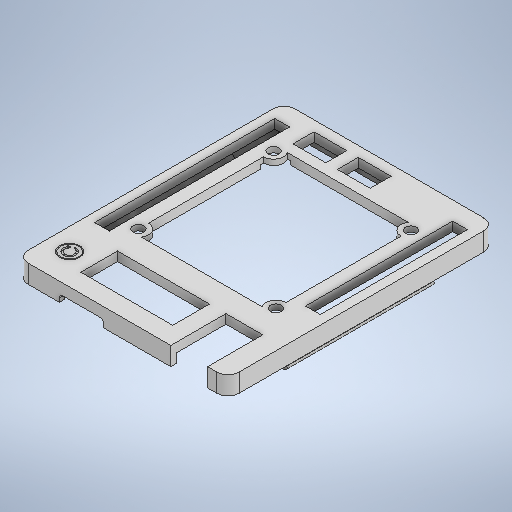
# Autodesk Inventor part: uno_r4_lid
Saved by Autodesk Inventor 2025.2 (Build 292293000, 293)
## iProperties
Created: 2025-03-24
Part Number: uno_r4_lid
Material: Generic
Document SubType Name: Modeling
Designer: caomi
Density: 1 g/cm^3
Appearance: Default
Author: caomi
Autodesk Inventor part; units mm, degrees
sketch "Sketch1" plane through (0, 0, 0) normal (0, 1, 0) x (-1, 0, 0)
  line L0 (0, 0) -> (53.34, 0) construction
  line L1 (53.34, 0) -> (53.34, -68.58) construction
  line L2 (53.34, -68.58) -> (0, -68.58) construction
  line L3 (0, -68.58) -> (0, 0) construction
  line L4 (55.34, -70.58) -> (55.34, 2)
  line L5 (55.34, 2) -> (-2, 2)
  line L6 (-2, 2) -> (-2, -70.58)
  line L7 (-2, -70.58) -> (55.34, -70.58)
  dimension "d0" = 53.34
  dimension "d1" = 68.58
  dimension "d2" = 2
  constraints: 16 end point, 4 parallel, 2 perpendicular, 1 horizontal, 3 other
  measures "d0" distance of L0.start L0.end
  measures "d1" distance of L2.end L0.start
  measures "d2" distance between parallel lines of L1 L4
extrude "Body" add sketch "Sketch1" against normal blind 5
fillet "Fillet1" radius 3 4 edges at (-55.34, -2.5, 2) (-55.34, -2.5, -70.58) (2, -2.5, -70.58) (2, -2.5, 2)
shell "Shell1" thickness 1.5 removed faces 1 at (-17.1133, -5, -45.3867)
sketch "Sketch2" plane through (0, -5, 0) normal (0, -1, 0) x (1, 0, 0)
  line L0 (-53.34, 0) -> (-53.34, -68.58) construction
  line L1 (-52.34, 0.5) -> (-1, 0.5) projected
  line L2 (-1, 2) -> (-52.34, 2) projected
  line L3 (-43.84, 0.5) -> (-31.84, 0.5)
  line L4 (-31.84, 0.5) -> (-31.84, 2)
  line L5 (-31.84, 2) -> (-43.84, 2)
  line L6 (-43.84, 2) -> (-43.84, 0.5)
  line L7 (-13.54, 2) -> (-3.54, 2)
  line L8 (-3.54, 2) -> (-3.54, -13)
  line L9 (-3.54, -13) -> (-13.54, -13)
  line L10 (-13.54, -13) -> (-13.54, 2)
  dimension "d8" = 12
  dimension "d15" = 9.5
  dimension "d16" = 39.8
  dimension "d17" = 10
  dimension "d18" = 15
  constraints: 16 end point, 4 parallel, 3 point on line, 2 horizontal, 2 perpendicular
  measures "d8" distance between parallel lines of L4 L6
  measures "d15" distance from line of L0 L5.end
  measures "d16" distance between parallel lines of L0 L10
  measures "d17" distance between parallel lines of L8 L10
  measures "d18" distance of L9.end L7.start
extrude "USB-C port" cut sketch "Sketch2" against normal blind 2 contours L6 L2 L4 L1
fillet "Fillet2" radius 1 2 edges at (-43.84, -3, 1.25) (-31.84, -3, 1.25)
extrude "DC jack port" cut sketch "Sketch2" against normal through all contours L10 L2 L8 L1 | L1 L8 L9 L10
sketch "Sketch3" plane through (0, 0, 0) normal (0, 1, 0) x (1, 0, 0)
  line L0 (-53.34, 0) -> (-53.34, 68.58) construction
  line L1 (-52.84, 65.58) -> (-48.84, 65.58)
  line L2 (-48.84, 65.58) -> (-48.84, 16.58)
  line L3 (-48.84, 16.58) -> (-52.84, 16.58)
  line L4 (-52.84, 16.58) -> (-52.84, 65.58)
  line L5 (-53.34, 68.58) -> (0, 68.58) construction
  line L6 (-0.5, 65.58) -> (-4.5, 65.58)
  line L7 (-4.5, 65.58) -> (-4.5, 25.58)
  line L8 (-4.5, 25.58) -> (-0.5, 25.58)
  line L9 (-0.5, 25.58) -> (-0.5, 65.58)
  line L10 (0, 68.58) -> (0, 0) construction
  line L11 (-32.34, 67.78) -> (-23.44, 67.78)
  line L12 (-23.44, 67.78) -> (-23.44, 62.08)
  line L13 (-23.44, 62.08) -> (-32.34, 62.08)
  line L14 (-32.34, 62.08) -> (-32.34, 67.78)
  dimension "d19" = 0.5
  dimension "d20" = 4
  dimension "d23" = 3
  dimension "d24" = 52
  dimension "d25" = 0.5
  dimension "d26" = 3
  dimension "d27" = 40
  dimension "d28" = 21
  dimension "d29" = 8.9
  dimension "d30" = 5.7
  dimension "d31" = 0.8
  constraints: 24 end point, 6 parallel, 3 horizontal, 3 perpendicular, 1 collinear
  measures "d19" distance between parallel lines of L0 L4
  measures "d20" distance of L2.end L3.end
  measures "d23" distance between parallel lines of L5 L1
  measures "d24" distance between parallel lines of L3 L5
  measures "d25" distance between parallel lines of L10 L9
  measures "d26" distance from line of L5 L6.start
  measures "d27" distance of L8.end L6.start
  measures "d28" distance from line of L0 L11.start
  measures "d29" distance of L11.start L11.end
  measures "d30" distance of L13.end L11.start
  measures "d31" vertical distance of L0.end L11.start
extrude "GPIO cutouts" cut sketch "Sketch3" against normal blind 5
sketch "Sketch4" plane through (0, 0, 0) normal (0, 1, 0) x (1, 0, 0)
  line L0 (-48.17, 60.8905) -> (-5.17, 60.8905) construction
  line L1 (-5.17, 60.8905) -> (-5.17, 17.8905) construction
  line L2 (-5.17, 17.8905) -> (-48.17, 17.8905) construction
  line L3 (-48.17, 17.8905) -> (-48.17, 60.8905) construction
  line L4 (-48.17, 60.8905) -> (-5.17, 17.8905) construction
  line L5 (-5.17, 60.8905) -> (-48.17, 17.8905) construction
  line L6 (-45.36, 57.7615) -> (-7.98, 57.7615) construction
  line L7 (-7.98, 57.7615) -> (-7.98, 21.0195) construction
  line L8 (-7.98, 21.0195) -> (-45.36, 21.0195) construction
  line L9 (-45.36, 21.0195) -> (-45.36, 57.7615) construction
  line L10 (-45.36, 57.7615) -> (-7.98, 21.0195) construction
  line L11 (-7.98, 57.7615) -> (-45.36, 21.0195) construction
  circle A0 centre (-7.98, 21.0195) radius 1.5
  circle A1 centre (-45.36, 21.0195) radius 1.5
  circle A2 centre (-45.36, 57.7615) radius 1.5
  circle A3 centre (-7.98, 57.7615) radius 1.5
  circle A4 centre (-7.98, 21.0195) radius 2.75
  circle A5 centre (-45.36, 21.0195) radius 2.75
  circle A6 centre (-7.98, 57.7615) radius 2.75
  circle A7 centre (-45.36, 57.7615) radius 2.75
  line L12 (-10.73, 21.0195) -> (-42.61, 21.0195)
  line L13 (-45.36, 23.7695) -> (-45.36, 55.0115)
  line L14 (-42.61, 57.7615) -> (-10.73, 57.7615)
  line L15 (-7.98, 23.7695) -> (-7.98, 55.0115)
  line L16 (-4.5, 65.58) -> (-0.5, 65.58) projected
  line L17 (-48.84, 65.58) -> (-4.5, 65.58) construction
  line L18 (-43.0551, 59.2615) -> (-10.2849, 59.2615)
  line L19 (-43.0551, 19.5195) -> (-10.2849, 19.5195)
  point P0 (-26.67, 39.3905)
  point P1 (-26.67, 65.58)
  dimension "d34" = 43
  dimension "d35" = 37.38
  dimension "d36" = 36.742
  dimension "d37" = 3
  dimension "d43" = 5.5
  dimension "d101" = 1.5
  dimension "d102" = 1.5
  constraints: 38 end point, 12 point on circle, 8 centre point, 8 coincident, 7 point on line, 6 equal radius, 6 parallel, 5 midpoint, 3 collinear, 3 perpendicular, 2 horizontal, 1 vertical alignment
  measures "d34" distance of L1.end L2.end
  measures "d35" distance of L7.end L8.end
  measures "d36" distance of L8.end L6.start
  measures "d37" diameter of A0
  measures "d43" diameter of A4
  measures "d101" distance between parallel lines of L14 L18
  measures "d102" distance between parallel lines of L12 L19
sketch "Sketch7" plane through (-52.34, -1.5, -69.08) normal (0, -1, 0) x (1, 0, 0)
  line L0 (3.5, 52.5) -> (3.5, 3.5) projected
  line L1 (3.5, 3.5) -> (-0.5, 3.5) projected
  line L2 (-0.5, 3.5) -> (-0.5, 52.5) projected
  line L3 (-0.5, 52.5) -> (3.5, 52.5) projected
  line L4 (47.84, 43.5) -> (51.84, 43.5) projected
  line L5 (51.84, 43.5) -> (51.84, 3.5) projected
  line L6 (51.84, 3.5) -> (47.84, 3.5) projected
  line L7 (47.84, 3.5) -> (47.84, 43.5) projected
  line L8 (28.9, 7) -> (28.9, 1.3) projected
  line L9 (28.9, 1.3) -> (20, 1.3) projected
  line L10 (20, 1.3) -> (20, 7) projected
  line L11 (20, 7) -> (28.9, 7) projected
  line L12 (48.8, 69.58) -> (48.8, 56.08) projected
  line L13 (48.8, 56.08) -> (38.8, 56.08) projected
  line L14 (38.8, 56.08) -> (38.8, 69.58) projected
  line L15 (0, 69.58) -> (38.8, 69.58) projected
  arc A0 (0, 69.58) -> (-1.5, 68.08) centre (0, 68.08) ccw projected
  line L16 (-1.5, 1.5) -> (-1.5, 68.08) projected
  arc A1 (-1.5, 1.5) -> (0, 0) centre (0, 1.5) ccw projected
  line L17 (51.34, 0) -> (0, 0) projected
  arc A2 (51.34, 0) -> (52.84, 1.5) centre (51.34, 1.5) ccw projected
  line L18 (52.84, 68.08) -> (52.84, 1.5) projected
  arc A3 (52.84, 68.08) -> (51.34, 69.58) centre (51.34, 68.08) ccw projected
  line L19 (48.8, 69.58) -> (51.34, 69.58) projected
  point P0 (52.34, 69.08)
extrude "Thicken the top" add sketch "Sketch7" along normal blind 1
extrude "Screw hole motor driver" cut sketch "Sketch4" against normal through all contours A0 | A1 | A2 | A3
sketch "Sketch5" plane through (-52.34, -2.5, -69.08) normal (0, -1, 0) x (1, 0, 0)
  line L0 (47.51, 46.2419) -> (44.36, 44.4232)
  line L1 (44.36, 44.4232) -> (41.21, 46.2419)
  line L2 (41.21, 46.2419) -> (41.21, 49.8792)
  line L3 (41.21, 49.8792) -> (44.36, 51.6978)
  line L4 (44.36, 51.6978) -> (47.51, 49.8792)
  line L5 (47.51, 49.8792) -> (47.51, 46.2419)
  line L6 (47.51, 13.1372) -> (47.51, 9.4999)
  line L7 (47.51, 9.4999) -> (44.36, 7.6812)
  line L8 (44.36, 7.6812) -> (41.21, 9.4999)
  line L9 (41.21, 9.4999) -> (41.21, 13.1372)
  line L10 (41.21, 13.1372) -> (44.36, 14.9558)
  line L11 (44.36, 14.9558) -> (47.51, 13.1372)
  circle A0 centre (6.98, 48.0605) radius 1.5 projected
  line L12 (10.13, 49.8792) -> (10.13, 46.2419)
  line L13 (10.13, 46.2419) -> (6.98, 44.4232)
  line L14 (6.98, 44.4232) -> (3.83, 46.2419)
  line L15 (3.83, 46.2419) -> (3.83, 49.8792)
  line L16 (3.83, 49.8792) -> (6.98, 51.6978)
  line L17 (6.98, 51.6978) -> (10.13, 49.8792)
  line L18 (10.13, 13.1372) -> (10.13, 9.4999)
  line L19 (10.13, 9.4999) -> (6.98, 7.6812)
  line L20 (6.98, 7.6812) -> (3.83, 9.4999)
  line L21 (3.83, 9.4999) -> (3.83, 13.1372)
  line L22 (3.83, 13.1372) -> (6.98, 14.9558)
  line L23 (6.98, 14.9558) -> (10.13, 13.1372)
  circle A1 centre (6.98, 11.3185) radius 1.5 projected
  circle A2 centre (44.36, 11.3185) radius 1.5 projected
  circle A3 centre (44.36, 48.0605) radius 1.5 projected
  circle A4 centre (6.98, 48.0605) radius 1.5 projected
  dimension "d40" = 6.3
  constraints: 48 end point, 5 coincident, 4 vertical, 3 equal length, 52 other
  measures "d40" distance between parallel lines of L2 L5
extrude "M3 nut slot" cut sketch "Sketch5" against normal blind 1 contours L0 L1 L2 L3 L4 L5 | L6 L7 L8 L9 L10 L11 | L12 L13 L14 L15 L16 L17 | L18 L19 L20 L21 L22 L23 | A1 | A2 | A3
extrude "Recess face motor driver" cut sketch "Sketch4" against normal blind 3 contours A4 L12 A5 L13 A7 L14 A6 L15 | L19 A5 L12 A4 | L14 A7 L18 A6
ref_plane "Work Plane1" through (0, 0, -15) normal (0, 0, 1) x (1, 0, 0)
ref_plane "Work Plane2" through (0, 0, -55) normal (0, 0, 1) x (1, 0, 0)
sketch "Sketch8" plane through (0, 0, -15) normal (0, 0, 1) x (1, 0, 0)
  line L0 (-53.84, -3.5) -> (-52.64, -4.7)
  line L1 (-52.64, -4.7) -> (-52.64, -7.3)
  line L2 (-52.64, -7.3) -> (-53.84, -7.3)
  line L3 (-53.84, -7.3) -> (-53.84, -3.5)
  line L4 (-53.84, -2.5) -> (-53.84, -5) projected
  line L5 (-53.84, -5.7) -> (-54.64, -6.5)
  line L6 (-54.64, -6.5) -> (-53.84, -7.3)
  line L7 (-54.64, -6.5) -> (-53.84, -6.5) construction
  point P0 (0, 0)
  point P1 (-53.84, -7.5)
  dimension "d53" = 1.5
  dimension "d54" = 45
  dimension "d56" = 1.2
  dimension "d57" = 45
  dimension "d58" = 0.8
  dimension "d62" = 1.5
  constraints: 15 end point, 2 perpendicular, 2 point on line, 2 vertical, 1 collinear, 1 other
  measures "d53" distance of L4.end L0.start
  measures "d54" angle of L0 L4
  measures "d56" distance of L2.end L1.end
  measures "d57" angle of L3 L6
  measures "d58" distance of L5.end L7.end
  measures "d62" distance from line of L4.end L7
extrude "Snap tab 1" add sketch "Sketch8" against normal up to surface (40 mm away)
fillet "Fillet3" radius 0.5 1 edges at (-54.64, -6.5, -35)
ref_plane "Work Plane3" through (-26.67, 0, -67.58) normal (-1, 0, 0) x (0, 0, 1)
mirror "Snap tab right side" about plane through (-26.67, 0, -67.58) normal (-1, 0, 0) of "Snap tab 1", "Fillet3"
sketch "Sketch9" plane through (-52.34, -2.5, -69.08) normal (0, -1, 0) x (1, 0, 0)
  line L0 (52.34, 69.08) -> (-1, 69.08) construction
  line L1 (-1, 69.08) -> (-1, 0.5) construction
  circle A0 centre (2.937, 62.73) radius 2.5
  circle A1 centre (2.937, 62.73) radius 2.75
  dimension "d66" = 6.35
  dimension "d67" = 3.937
  dimension "d71" = 5
  dimension "d73" = 5.5
  constraints: 2 centre point, 2 coincident
  measures "d66" distance from line of L0 point (2.937, 62.73)
  measures "d67" distance from line of L1 point (2.937, 62.73)
  measures "d71" diameter of A0
  measures "d73" diameter of A1
extrude "Extrusion12" cut sketch "Sketch9" against normal through all contours A0 | A1
extrude "Reset button" add sketch "Sketch9" along normal blind 3 and the other way blind 2.5 separate body contours A0
ref_plane "Work Plane5" through (-49.403, -2.5, -6.35) normal (0, 0, 1) x (1, 0, 0)
ref_plane "Work Plane4" through (-49.403, -2.5, -8.85) normal (0, 0, 1) x (1, 0, 0)
sketch "Sketch10" plane through (-49.403, -2.5, -6.35) normal (0, 0, 1) x (1, 0, 0)
  line L0 (-2.5, 2.5) -> (-2.5, -3) projected
  line L1 (-2.5, -2.1) -> (-3.3, -1.3)
  line L2 (-3.3, -1.3) -> (-2.5, -0.5)
  line L3 (-3.3, -1.3) -> (-2.5, -1.3) construction
  line L4 (2.75, 0) -> (-2.75, 0) projected
  line L5 (-2.75, 0) -> (-2.75, 0.65)
  line L6 (-2.75, 0.65) -> (-3.7, -0.3)
  line L7 (-2.75, -2.25) -> (-2.75, -3.25)
  line L8 (-4.25, -3.25) -> (-4.25, 0)
  line L9 (-3.7, -0.3) -> (-3.7, -1.3)
  line L10 (-3.7, -1.3) -> (-2.75, -2.25)
  line L11 (-2.75, 0) -> (-4.25, 0)
  line L12 (-2.5, -2.1) -> (-2.5, -0.5)
  line L13 (-2.5, -3) -> (2.5, -3) projected
  line L14 (0, -4.6511) -> (0, -1.8) construction
  line L15 (-4.25, -3.25) -> (-2.75, -3.25)
  point P0 (49.403, 2.5)
  point P1 (0, -3)
  point P2 (-3.4, 0)
  dimension "d79" = 45
  dimension "d80" = 0.8
  dimension "d81" = 0.5
  dimension "d82" = 135
  dimension "d83" = 1
  dimension "d85" = 1.5
  dimension "d90" = 1
  dimension "d98" = 0.4
  constraints: 26 end point, 5 point on line, 5 vertical, 2 collinear, 2 horizontal, 1 midpoint, 1 parallel, 1 perpendicular, 1 other
  measures "d79" angle of L0 L2
  measures "d80" distance of L1.end L3.end
  measures "d81" vertical distance of L2.end L4.end
  measures "d82" angle of L5 L6
  measures "d83" distance of L6.end L9.end
  measures "d85" distance from line of L4.end L8
  measures "d90" distance of L7.start L7.end
  measures "d98" distance from line of L1.end L9
revolve "Revolution1" add sketch "Sketch10" angle 360 about axis through (-49.403, -7.1511, -6.35) along (0, 1, 0) bodies 2 contours L0 L1 L2
revolve "Revolution3" cut sketch "Sketch10" angle 360 about axis through (-49.403, -7.1511, -6.35) along (0, 1, 0) bodies 1 contours L11 L6 L5
revolve "Revolution2" add sketch "Sketch10" angle 360 about axis through (-49.403, -7.1511, -6.35) along (0, 1, 0) bodies 1 contours L6 L9 L10 L7 L15 L8 L11
fillet "Fillet5" radius 1 1 edges at (-45.153, -5.75, -6.35)
ref_plane "Work Plane6" through (-49.403, 0.5, -6.35) normal (0, 1, 0) x (1, 0, 0)
sketch "Sketch11" plane through (-49.403, 0, -6.35) normal (0, 1, 0) x (1, 0, 0)
  arc A0 (-1.0607, 1.0607) -> (0, 1.5) centre (0, 0) ccw construction
  arc A1 (-1.2021, 1.2021) -> (0, 1.7) centre (0, 0) ccw
  arc A2 (-0.9192, 0.9192) -> (0, 1.3) centre (0, 0) ccw
  arc A3 (-0.9192, 0.9192) -> (-1.2021, 1.2021) centre (-1.0607, 1.0607) ccw
  arc A4 (0, 1.7) -> (0, 1.3) centre (0, 1.5) ccw
  line L0 (0, 0) -> (-1.0607, 1.0607) construction
  line L1 (0, 0) -> (0, 1.5) construction
  line L2 (-1.0607, 1.0607) -> (-1.5607, 1.0607) construction
  line L3 (-1.0607, 1.2607) -> (-1.5607, 1.2607)
  line L4 (-1.5607, 0.8607) -> (-1.0607, 0.8607)
  arc A5 (-1.0607, 0.8607) -> (-1.0607, 1.2607) centre (-1.0607, 1.0607) ccw
  arc A6 (-1.5607, 1.2607) -> (-1.5607, 0.8607) centre (-1.5607, 1.0607) ccw
  line L5 (-1.0607, 1.0607) -> (-1.0607, 0.5607) construction
  line L6 (-1.2607, 1.0607) -> (-1.2607, 0.5607)
  line L7 (-0.8607, 0.5607) -> (-0.8607, 1.0607)
  arc A7 (-0.8607, 1.0607) -> (-1.2607, 1.0607) centre (-1.0607, 1.0607) ccw
  arc A8 (-1.2607, 0.5607) -> (-0.8607, 0.5607) centre (-1.0607, 0.5607) ccw
  circle A9 centre (0, 0) radius 2.5 projected
  point P0 (49.403, -6.35)
  point P1 (-1.3107, 1.0607)
  point P2 (-1.0607, 0.8107)
  point P3 (-1.466, 0.8607)
  point P4 (-1.2223, 0.4428)
  point P5 (-0.8607, 1.0607)
  point P6 (-1.0607, 1.2607)
  dimension "d91" = 1.5
  dimension "d92" = 45
  dimension "d93" = 0.4
  dimension "d94" = 0.5
  dimension "d95" = 0.5
  constraints: 20 end point, 19 point on circle, 12 tangent, 9 centre point, 2 concentric, 2 midpoint, 2 parallel, 1 coincident, 1 horizontal, 1 perpendicular, 1 vertical
  measures "d91" radius of A0
  measures "d92" angle of L1 L0
  measures "d93" diameter of A3
  measures "d94" distance of L0.end L2.end
  measures "d95" distance of L0.end L5.end
extrude "Extrusion14" cut sketch "Sketch11" against normal blind 0.5 contours A7 L6 L4 A1 | A1 L4 A6 L3 A3 | A3 A5 L4 L6 A7 | L4 L6 A8 A2 A4 A1 | L4 A5 A2 A8 L6 | L7 A8 A2 A3 bodies 2
fillet "Fillet6" radius 0.5 1 edges at (-46.103, -3.8, -6.35)
sketch "Sketch12" plane through (0, 0, 0) normal (0, 1, 0) x (1, 0, 0)
  line L0 (-43.0261, 13) -> (-18.0261, 13)
  line L1 (-18.0261, 13) -> (-18.0261, 3)
  line L2 (-18.0261, 3) -> (-43.0261, 3)
  line L3 (-43.0261, 3) -> (-43.0261, 13)
  line L4 (-13.54, 13) -> (-3.54, 13) projected
  line L5 (-35.4833, 62.08) -> (-44.3833, 62.08)
  line L6 (-44.3833, 62.08) -> (-44.3833, 67.78)
  line L7 (-44.3833, 67.78) -> (-35.4833, 67.78)
  line L8 (-35.4833, 67.78) -> (-35.4833, 62.08)
  line L9 (-23.44, 62.08) -> (-32.34, 62.08) projected
  line L10 (-32.34, 67.78) -> (-23.44, 67.78) projected
  point P0 (0, 0)
  dimension "d105" = 10
  dimension "d106" = 25
  constraints: 16 end point, 4 collinear, 4 parallel, 2 horizontal, 2 perpendicular
  measures "d105" distance of L2.end L0.start
  measures "d106" distance of L1.end L2.end
extrude "Extrusion15" cut sketch "Sketch12" against normal blind 3 bodies 1
equation "\"d2\" = base_wall + tolerance_general"
equation "\"d6\" = base_wall"
equation "\"uno_width\" = 53.34"
equation "\"uno_length\" = 68.58"
equation "\"base_wall\" = 1.5"
equation "\"tolerance_general\" = 0.5"
body "Solid1"
body "Solid2"
